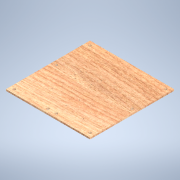
# Autodesk Inventor part: grounplate
Saved by Autodesk Inventor 2020 (Build 240168000, 168)
## iProperties
Created: 2021-02-27
Part Number: grounplate
Material: Wood (Birch)
Document SubType Name: Modeling
Designer: Bernard Li
Density: 0.55 g/cm^3
Appearance: Birch - Natural Polished
Author: Bernard Li
Autodesk Inventor part; units mm, degrees
ref_plane "YZ Plane" through (0, 0, 0) normal (1, 0, 0) x (0, 1, 0)
ref_plane "XZ Plane" through (0, 0, 0) normal (0, 1, 0) x (-1, 0, 0)
ref_plane "XY Plane" through (0, 0, 0) normal (0, 0, 1) x (1, 0, 0)
sketch "Sketch1" plane through (0, 0, 0) normal (0, 1, 0) x (-1, 0, 0)
  line L0 (101.6, 0) -> (-101.6, 0)
  line L1 (-101.6, 0) -> (-101.6, -203.2)
  line L2 (-101.6, -203.2) -> (101.6, -203.2)
  line L3 (101.6, -203.2) -> (101.6, 0)
  dimension "d0" = 203.2
  dimension "d1" = 203.2
  constraints: 8 end point, 2 parallel, 1 horizontal, 1 perpendicular
  measures "d0" distance of L2.end L1.end
  measures "d1" distance of L1.end L0.end
extrude "Extrusion1" add sketch "Sketch1" along normal blind 3.81
sketch "Sketch2" plane through (0, 3.81, 0) normal (0, 1, 0) x (1, 0, 0)
  circle A0 centre (-91.44, 10.16) radius 10.16
  circle A1 centre (-91.44, 10.16) radius 3.175
  line L0 (-101.6, 203.2) -> (-101.6, 0) projected
  line L1 (-101.6, 101.6) -> (101.6, 101.6)
  line L2 (101.6, 0) -> (101.6, 203.2) projected
  line L3 (-101.6, 0) -> (101.6, 0) projected
  line L4 (0, 0) -> (0, 101.6)
  circle A2 centre (91.44, 10.16) radius 10.16
  circle A3 centre (91.44, 10.16) radius 3.175
  circle A4 centre (-91.44, 193.04) radius 10.16
  circle A5 centre (-91.44, 193.04) radius 3.175
  circle A6 centre (91.44, 193.04) radius 10.16
  circle A7 centre (91.44, 193.04) radius 3.175
  point P0 (0, 0)
  dimension "d4" = 20.32
  dimension "d5" = 6.35
  constraints: 8 centre point, 6 symmetric about line, 4 coincident, 4 end point, 3 midpoint, 1 tangent, 9 other
  measures "d4" diameter of A0
  measures "d5" diameter of A1
extrude "Extrusion2" cut sketch "Sketch2" against normal blind 3.81 contours A1 | A3 | A5 | A7
sketch "Sketch3" plane through (0, 3.81, 0) normal (0, 1, 0) x (1, 0, 0)
  line L0 (101.6, 0) -> (101.6, 203.2) projected
  line L1 (101.6, 101.6) -> (-101.6, 101.6)
  line L2 (-101.6, 203.2) -> (-101.6, 0) projected
  circle A0 centre (-91.44, 111.76) radius 10.16
  circle A1 centre (-91.44, 111.76) radius 3.175
  circle A2 centre (91.44, 111.76) radius 10.16
  circle A3 centre (91.44, 111.76) radius 3.175
  point P0 (-100.0125, 103.1875)
  dimension "d8" = 20.32
  dimension "d9" = 6.35
  dimension "d10" = 20.32
  dimension "d11" = 6.35
  constraints: 4 centre point, 4 tangent, 2 coincident, 2 end point, 2 midpoint
  measures "d8" diameter of A0
  measures "d9" diameter of A1
  measures "d10" diameter of A2
  measures "d11" diameter of A3
extrude "Extrusion3" cut sketch "Sketch3" against normal blind 3.81 contours A1 | A3
sketch "Sketch4" plane through (0, 3.81, 0) normal (0, 1, 0) x (1, 0, 0)
  circle A0 centre (-48.895, 113.03) radius 1.5
  circle A1 centre (-48.895, 113.03) radius 1.5
  circle A2 centre (-8.255, 113.03) radius 1.5
  circle A3 centre (-8.255, 113.03) radius 1.5
  line L0 (-3.175, 107.95) -> (-13.335, 107.95)
  line L1 (-53.975, 130.175) -> (-53.975, 107.95)
  line L2 (-3.175, 107.95) -> (-53.975, 107.95)
  line L3 (-53.975, 107.95) -> (-53.975, 132.715)
  line L4 (-53.975, 132.715) -> (-3.175, 132.715)
  line L5 (-3.175, 132.715) -> (-3.175, 107.95)
  line L6 (-101.6, 203.2) -> (-101.6, 0) projected
  line L7 (101.6, 0) -> (101.6, 203.2) projected
  line L8 (-101.6, 0) -> (101.6, 0)
  line L9 (101.6, 0) -> (101.6, 107.95)
  line L10 (101.6, 107.95) -> (-101.6, 107.95)
  line L11 (-101.6, 107.95) -> (-101.6, 0)
  line L12 (-53.975, 120.3325) -> (-3.175, 120.3325)
  circle A4 centre (-48.895, 127.635) radius 1.5
  circle A5 centre (-48.895, 127.635) radius 1.5
  circle A6 centre (-8.255, 127.635) radius 1.5
  circle A7 centre (-8.255, 127.635) radius 1.5
  line L13 (-48.895, 107.95) -> (-48.895, 113.03)
  line L14 (-8.255, 107.95) -> (-8.255, 113.03)
  line L15 (-8.255, 132.715) -> (-8.255, 127.635)
  line L16 (-48.895, 132.715) -> (-48.895, 127.635)
  dimension "d14" = 107.95
  constraints: 30 end point, 8 centre point, 4 coincident, 4 parallel, 4 point on line, 4 symmetric about line, 4 vertical, 3 perpendicular, 2 midpoint, 1 collinear, 4 other
  measures "d14" distance of L9.end L7.start
extrude "Extrusion4" cut sketch "Sketch4" against normal blind 3.81 contours A0 | A2 | A6 | A4
sketch "Sketch5" plane through (0, 3.81, 0) normal (0, 1, 0) x (1, 0, 0)
  circle A0 centre (10.16, 10.16) radius 10.16
  circle A1 centre (10.16, 10.16) radius 3.175
  line L0 (-101.6, 0) -> (101.6, 0) projected
  line L1 (101.6, 203.2) -> (-101.6, 203.2) projected
  line L2 (0, 203.2) -> (0, 150.8125)
  circle A2 centre (-10.16, 10.16) radius 10.16
  circle A3 centre (-10.16, 10.16) radius 3.175
  dimension "d17" = 20.32
  dimension "d18" = 6.35
  constraints: 4 centre point, 2 coincident, 2 end point, 2 symmetric about line, 2 tangent, 1 midpoint, 1 vertical, 2 other
  measures "d17" diameter of A0
  measures "d18" diameter of A1
extrude "Extrusion5" cut sketch "Sketch5" against normal blind 3.81 contours A1 | A3
sketch "Sketch6" plane through (0, 3.81, 0) normal (0, 1, 0) x (1, 0, 0)
  line L0 (-44.1448, 101.6) -> (0, 101.6)
  line L1 (0, 101.6) -> (0, 136.525)
  line L2 (0, 136.525) -> (-44.1448, 136.525)
  line L3 (-44.1448, 136.525) -> (-44.1448, 101.6)
  circle A0 centre (-40.1448, 132.5875) radius 1.5
  circle A1 centre (-40.1448, 132.5875) radius 1.5
  circle A2 centre (-40.1448, 105.5375) radius 1.5
  circle A3 centre (-40.1448, 105.5375) radius 1.5
  circle A4 centre (-4, 105.5375) radius 1.5
  circle A5 centre (-4, 105.5375) radius 1.5
  circle A6 centre (-4, 132.5875) radius 1.5
  circle A7 centre (-4, 132.5875) radius 1.5
  line L4 (-101.6, 203.2) -> (-101.6, 0) projected
  line L5 (-101.6, 101.6) -> (101.6, 101.6)
  line L6 (101.6, 0) -> (101.6, 203.2) projected
  constraints: 10 end point, 8 centre point, 4 coincident, 2 midpoint, 2 parallel, 1 horizontal, 1 perpendicular
extrude "Extrusion6" cut sketch "Sketch6" against normal blind 3.81 contours A0 | A2 | A4 | A6
sketch "Sketch7" plane through (0, 3.81, 0) normal (0, 1, 0) x (1, 0, 0)
  circle A0 centre (2.54, 15.24) radius 1.5875
  circle A1 centre (2.54, 15.24) radius 1.5875
  circle A2 centre (50.8, 13.97) radius 1.5875
  circle A3 centre (45.72, 66.04) radius 1.5875
  circle A4 centre (17.78, 66.04) radius 1.5875
  circle A5 centre (50.8, 13.97) radius 1.5875
  line L0 (50.8, 13.97) -> (50.8, 0)
  line L1 (0, 0) -> (53.34, 0)
  line L2 (50.8, 0) -> (53.34, 0)
  line L3 (53.34, 0) -> (53.34, 66.04)
  line L4 (53.34, 66.04) -> (53.34, 68.58)
  line L5 (53.34, 68.58) -> (0, 68.58)
  line L6 (0, 68.58) -> (0, 0)
  line L7 (0, 0) -> (53.34, 0)
  line L8 (2.54, 15.24) -> (0, 15.24)
  line L9 (0, 66.04) -> (0, 0)
  circle A6 centre (17.78, 66.04) radius 1.5875
  line L10 (17.78, 66.04) -> (17.78, 68.58)
  line L11 (45.72, 66.04) -> (45.72, 68.58)
  line L12 (23.5657, 188.7512) -> (23.5657, 202.7212)
  circle A7 centre (23.5657, 188.7512) radius 1.5875
  line L13 (23.5657, 202.7212) -> (21.0257, 202.7212)
  line L14 (74.3657, 202.7212) -> (21.0257, 202.7212)
  line L15 (74.3657, 202.7212) -> (21.0257, 202.7212)
  line L16 (74.3657, 136.6812) -> (74.3657, 202.7212)
  line L17 (74.3657, 134.1412) -> (74.3657, 202.7212)
  line L18 (21.0257, 202.7212) -> (21.0257, 136.6812)
  circle A8 centre (56.5857, 136.6812) radius 1.5875
  circle A9 centre (56.5857, 136.6812) radius 1.5875
  line L19 (56.5857, 136.6812) -> (56.5857, 134.1412)
  line L20 (21.0257, 134.1412) -> (74.3657, 134.1412)
  line L21 (28.6457, 136.6812) -> (28.6457, 134.1412)
  circle A10 centre (28.6457, 136.6812) radius 1.5875
  line L22 (21.0257, 136.6812) -> (21.0257, 134.1412)
  circle A11 centre (71.8257, 187.4812) radius 1.5875
  circle A12 centre (71.8257, 187.4812) radius 1.5875
  line L23 (71.8257, 187.4812) -> (74.3657, 187.4812)
  circle A13 centre (23.5657, 188.7512) radius 1.5875
  point P0 (71.8257, 187.4812)
  constraints: 48 end point, 14 centre point, 14 perpendicular, 8 coincident, 8 point on line, 2 parallel, 1 vertical
extrude "Extrusion7" cut sketch "Sketch7" against normal blind 3.81 contours A10 | A8 | A11 | A7
body "Solid1"
